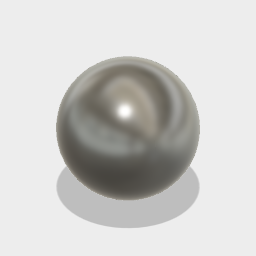
lever (Autodesk Fusion 360 design; units mm, degrees)
Autodesk Fusion 360 part; units mm, degrees
note: some values were not read from the file. Set by a fixed rule: which sketch regions a step uses.
sketch "スケッチ1" plane through (0, 0, 0) normal (1, 0, 0) x (0, 0, -1)
  line L0 (-1.75, 0) -> (-22.5, 0)
  line L1 (0, -20) -> (4.5, -20)
  line L2 (4.5, -20) -> (4.5, -30)
  line L3 (0, 1.75) -> (0, 22.5)
  line L4 (0, 20) -> (0, -20)
  arc A0 (4.5, -30) -> (0, 20) centre (-0.2225, -5.2225) ccw
  dimension "d4" = 4.5
  dimension "d8" = 40
  dimension "d10" = 10
  dimension "d12" = 25.2235
  measures "d4" distance of L1.end L1.start
  measures "d8" distance of L4.start L1.start
  measures "d10" distance of L1 L2.end
  measures "d12" radius of A0
revolve "回転2" add sketch "スケッチ1" angle 360 about axis through (0, 20, 0) along (0, -1, 0)
